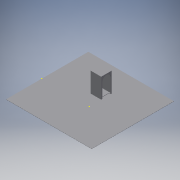
# Autodesk Inventor part: mock ground
Saved by Autodesk Inventor 2019 (Build 230136000, 136)
## iProperties
Created: 2019-11-06
Part Number: mock ground
Material: Generic
Document SubType Name: Modeling
Designer: Administrator
Density: 1 g/cm^3
Appearance: Default
Author: Administrator
Autodesk Inventor part; units mm, degrees
ref_plane "YZ Plane" through (0, 0, 0) normal (1, 0, 0) x (0, 1, 0)
ref_plane "XZ Plane" through (0, 0, 0) normal (0, 1, 0) x (-1, 0, 0)
ref_plane "XY Plane" through (0, 0, 0) normal (0, 0, 1) x (1, 0, 0)
sketch "Sketch1" plane through (0, 0, 0) normal (0, 1, 0) x (-1, 0, 0)
  line L0 (-5191.4732, 4324.9541) -> (11502.4171, 4324.9541)
  line L1 (11502.4171, 4324.9541) -> (11502.4171, -7800.5964)
  line L2 (11502.4171, -7800.5964) -> (-5191.4732, -7800.5964)
  line L3 (-5191.4732, -7800.5964) -> (-5191.4732, 4324.9541)
  constraints: 8 end point
extrude "Extrusion1" add sketch "Sketch1" along normal blind 25.4
sketch "Sketch2" plane through (0, 0, 0) normal (0, -1, 0) x (1, 0, 0)
  circle A0 centre (-517.6476, -2116.7989) radius 63.5
  point P0 (0, 0)
  dimension "d2" = 127
  constraints: 1 centre point
  measures "d2" diameter of A0
extrude "Extrusion2" add sketch "Sketch2" along normal blind 228.6
sketch "Sketch3" plane through (0, 0, 0) normal (0, -1, 0) x (1, 0, 0)
  line L0 (-668.0718, -1421.9447) -> (601.9282, -1421.9447)
  line L1 (601.9282, -1421.9447) -> (601.9282, -2691.9447)
  line L2 (601.9282, -2691.9447) -> (-668.0718, -2691.9447)
  line L3 (-668.0718, -2691.9447) -> (-668.0718, -1421.9447)
  point P0 (0, 0)
  dimension "d5" = 1270
  dimension "d6" = 1270
  constraints: 8 end point, 2 parallel, 1 horizontal, 1 perpendicular
  measures "d5" distance of L1.end L2.end
  measures "d6" distance of L0.end L1.end
extrude "Extrusion3" add sketch "Sketch3" against normal blind 2413
sketch "Sketch4" plane through (601.9282, 25.4, -2691.9447) normal (1, 0, 0) x (0, 0, -1)
  point P0 (-2691.9447, -25.4)
sketch "Sketch5" plane through (601.9282, 25.4, -2691.9447) normal (1, 0, 0) x (0, 0, -1)
  line L0 (-7016.8988, 0) -> (5108.6517, 0) projected
  line L1 (-107.5467, 0) -> (-1123.5467, 0)
  line L2 (-1123.5467, 0) -> (-1123.5467, 1778)
  line L3 (-107.5467, 1778) -> (-107.5467, 0)
  arc A0 (-107.5467, 1778) -> (-1123.5467, 1778) centre (-615.5467, 1778) ccw
  line L4 (-1123.5467, 0) -> (-107.5467, 0)
  point P0 (-2691.9447, -25.4)
  constraints: 8 end point, 2 equal length, 2 point on circle, 2 tangent, 1 centre point, 1 horizontal, 1 perpendicular, 1 point on line
extrude "Extrusion4" cut sketch "Sketch5" against normal blind 198.374
sketch "Sketch7" plane through (0, 2413, 0) normal (0, 1, 0) x (1, 0, 0)
  line L0 (-638.7139, 1445.2256) -> (565.6407, 1445.2256)
  line L1 (565.6407, 1445.2256) -> (565.6407, 2663.1123)
  line L2 (565.6407, 2663.1123) -> (-638.7139, 2663.1123)
  line L3 (-638.7139, 2663.1123) -> (-638.7139, 1445.2256)
  point P0 (0, 0)
  constraints: 8 end point, 2 parallel, 1 horizontal, 1 perpendicular
extrude "Extrusion5" cut sketch "Sketch7" against normal blind 2349.5635
sketch "Sketch8" plane through (0, 2413, 0) normal (0, 1, 0) x (1, 0, 0)
  line L0 (601.9282, 2691.9447) -> (-668.0718, 2691.9447) projected
  line L1 (601.9282, 1568.398) -> (601.9282, 1421.9447) projected
  line L2 (-668.0718, 2691.9447) -> (601.9282, 2691.9447)
  line L3 (601.9282, 2691.9447) -> (601.9282, 1421.9447)
  line L4 (601.9282, 1421.9447) -> (-668.0718, 1421.9447)
  line L5 (-668.0718, 1421.9447) -> (-668.0718, 2691.9447)
  point P0 (0, 0)
  constraints: 8 end point, 2 parallel, 1 horizontal, 1 perpendicular
extrude "Extrusion6" add sketch "Sketch8" along normal blind 25.4
sketch "Sketch9" plane through (-11502.4171, 0, -7800.5964) normal (-1, 0, 0) x (0, 0, 1)
  point P0 (7800.5964, 0)
sketch "Sketch10" plane through (0, 25.4, 0) normal (0, 1, 0) x (1, 0, 0)
  line L0 (-5022.8081, 1131.8072) -> (-9439.699, 1131.8072)
  line L1 (-9439.699, 1131.8072) -> (-9439.699, 3378.3486)
  line L2 (-9439.699, 3378.3486) -> (-5022.8081, 3378.3486)
  line L3 (-5022.8081, 3378.3486) -> (-5022.8081, 1131.8072)
  point P0 (0, 0)
  constraints: 8 end point, 2 parallel, 1 horizontal, 1 perpendicular
extrude "Extrusion7" add sketch "Sketch10" along normal blind 2744.7875
sketch "Sketch11" plane through (-9439.699, 25.4, -1131.8072) normal (0, 0, 1) x (1, 0, 0)
  point P0 (9439.699, -25.4)
sketch "Sketch12" plane through (-9439.699, 25.4, -1131.8072) normal (0, 0, 1) x (1, 0, 0)
  line L0 (0, 0) -> (0, 2744.7875) projected
  line L1 (0, 2744.7875) -> (4416.8909, 2744.7875) projected
  line L2 (0, 2744.7875) -> (4416.8909, 2744.7875)
  line L3 (4416.8909, 2744.7875) -> (2411.6217, 4609.8649)
  line L4 (2411.6217, 4609.8649) -> (0, 2744.7875)
  point P0 (9439.699, -25.4)
  constraints: 6 end point, 1 collinear
extrude "Extrusion8" add sketch "Sketch12" against normal blind 2281.2375
body "Solid1"
